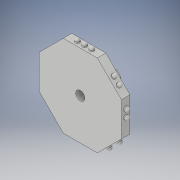
# Autodesk Inventor part: Right Braille Wheel
Saved by Autodesk Inventor 2017 (Build 210142000, 142)
## iProperties
Created: 2018-02-03
Part Number: Right Braille Wheel
Material: Generic
Document SubType Name: Modeling
Designer: Russ
Density: 1 g/cm^3
Appearance: Default
Author: Russ
Autodesk Inventor part; units mm, degrees
ref_plane "YZ Plane" through (0, 0, 0) normal (1, 0, 0) x (0, 1, 0)
ref_plane "XZ Plane" through (0, 0, 0) normal (0, 1, 0) x (-1, 0, 0)
ref_plane "XY Plane" through (0, 0, 0) normal (0, 0, 1) x (1, 0, 0)
sketch "Sketch1" plane through (0, 0, 0) normal (0, 0, 1) x (1, 0, 0)
  line L0 (6, 14.4853) -> (14.4853, 6)
  line L1 (14.4853, 6) -> (14.4853, -6)
  line L2 (14.4853, -6) -> (6, -14.4853)
  line L3 (6, -14.4853) -> (-6, -14.4853)
  line L4 (-6, -14.4853) -> (-14.4853, -6)
  line L5 (-14.4853, -6) -> (-14.4853, 6)
  line L6 (-14.4853, 6) -> (-6, 14.4853)
  line L7 (-6, 14.4853) -> (6, 14.4853)
  point P0 (0, 0)
  point P1 (0, 0)
  dimension "d2" = 12
  constraints: 16 end point, 1 coincident, 17 other
  measures "d2" distance of L4.end L5.end
extrude "Extrusion1" add sketch "Sketch1" along normal blind 3
sketch "Sketch2" plane through (-6, 14.4853, 0) normal (0, 1, 0) x (1, 0, 0)
  circle A0 centre (3.4656, -1.4986) radius 0.8
  circle A1 centre (6.0056, -1.4986) radius 0.8
  circle A2 centre (8.5456, -1.5014) radius 0.8
  line L0 (0, 0) -> (12, 0) projected
  line L1 (0, 0) -> (0, -3) projected
  line L2 (0, -3) -> (12, -3) projected
  line L3 (12, 0) -> (12, -3) projected
  point P0 (6, 0)
  dimension "d5" = 1.6
  dimension "d6" = 2.54
  dimension "d7" = 2.54
  dimension "d8" = 1.6
  dimension "d9" = 1.6
  dimension "d10" = 1.4986
  dimension "d24" = 1.4986
  dimension "d170" = 5.9944
  constraints: 3 centre point
  measures "d5" diameter of A0
  measures "d6" distance of A1.centre A0.centre
  measures "d7" distance of A2.centre A1.centre
  measures "d8" diameter of A1
  measures "d9" diameter of A2
  measures "d10" distance from line of L0 A1.centre
  measures "d24" distance from line of L2 A2.centre
  measures "d170" distance from line of L3 A1.centre
extrude "Extrusion2" add sketch "Sketch2" along normal blind 1.2 contours A0 | A1 | A2
fillet "Fillet1" radius 0.8 3 edges at (1.7456, 15.6853, 1.5014) (-0.7944, 15.6853, 1.4986) (-3.3344, 15.6853, 1.4986)
sketch "Sketch3" plane through (6, 14.4853, 0) normal (0.7071, 0.7071, 0) x (-0.7071, 0.7071, 0)
  circle A0 centre (-8.5456, 1.4986) radius 0.8
  circle A1 centre (-6.0056, 1.4986) radius 0.8
  circle A2 centre (-3.4656, 1.4986) radius 0.8
  line L0 (-10.0061, 2.6736) -> (-10.0061, 0)
  line L1 (-10.0061, 0) -> (0.0295, 0)
  line L2 (0, 3) -> (-12, 3) projected
  line L3 (-12, 0) -> (0, 0) projected
  line L4 (-12, 0) -> (-12, 3) projected
  point P0 (-3.9705, 2.6736)
  dimension "d25" = 1.6
  dimension "d26" = 2.54
  dimension "d27" = 2.54
  dimension "d28" = 1.6
  dimension "d29" = 1.6
  dimension "d31" = 1.4605
  dimension "d32" = 1.4986
  dimension "d34" = 0
  dimension "d35" = 1.4986
  dimension "d36" = 1.4986
  dimension "d169" = 5.9944
  constraints: 4 end point, 3 centre point
  measures "d25" diameter of A0
  measures "d26" distance of A1.centre A0.centre
  measures "d27" distance of A2.centre A1.centre
  measures "d28" diameter of A1
  measures "d29" diameter of A2
  measures "d31" distance from line of L0 A0.centre
  measures "d32" distance from line of L1 A2.centre
  measures "d34" distance between parallel lines of L3 L1
  measures "d35" distance from line of L1 A1.centre
  measures "d36" distance from line of L1 A0.centre
  measures "d169" distance from line of L4 A1.centre
sketch "Sketch4" plane through (14.4853, -6, 0) normal (1, 0, 0) x (0, 0, -1)
  circle A0 centre (-1.4986, 3.4544) radius 0.8
  circle A1 centre (-1.4986, 5.9944) radius 0.8
  circle A2 centre (-1.4986, 8.5344) radius 0.8
  line L0 (0.3264, 0) -> (0, 0)
  line L1 (0, 0) -> (0, 3.0295)
  line L2 (0, 3) -> (0, -5)
  line L3 (0, -5) -> (0, 3)
  line L4 (0, 12) -> (0, 0) projected
  line L5 (0, 0) -> (-3, 0) projected
  point P0 (0, 6)
  point P1 (0.3264, -0.9705)
  dimension "d40" = 1.6
  dimension "d41" = 2.54
  dimension "d42" = 2.54
  dimension "d43" = 1.6
  dimension "d44" = 1.6
  dimension "d46" = 1.4986
  dimension "d47" = 0
  dimension "d48" = 1.4986
  dimension "d49" = 1.4986
  dimension "d50" = 0
  dimension "d51" = 0
  dimension "d171" = 5.9944
  constraints: 8 end point, 3 centre point
  measures "d40" diameter of A0
  measures "d41" distance of A1.centre A0.centre
  measures "d42" distance of A2.centre A1.centre
  measures "d43" diameter of A1
  measures "d44" diameter of A2
  measures "d46" distance from line of L1 A2.centre
  measures "d47" distance between parallel lines of L3 L1
  measures "d48" distance from line of L1 A1.centre
  measures "d49" distance from line of L1 A0.centre
  measures "d50" distance between parallel lines of L4 L1
  measures "d51" distance between parallel lines of L5 L0
  measures "d171" distance from line of L5 A1.centre
sketch "Sketch6" plane through (-14.4853, -6, 0) normal (-1, 0, 0) x (0, 0, 1)
  circle A0 centre (1.5014, 3.4544) radius 0.8
  circle A1 centre (1.5014, 5.9944) radius 0.8
  circle A2 centre (1.5014, 8.5344) radius 0.8
  line L0 (1.3264, 0) -> (3, 0)
  line L1 (3, 0) -> (3, 4.0295)
  line L2 (3, -4) -> (3, 4)
  line L3 (0, 0) -> (0, 12) projected
  line L4 (3, 12) -> (3, 0) projected
  line L5 (0, 0) -> (3, 0) projected
  point P0 (0, 6)
  point P1 (1.3264, 0.0295)
  dimension "d70" = 1.6
  dimension "d71" = 2.54
  dimension "d72" = 2.54
  dimension "d73" = 1.6
  dimension "d74" = 1.6
  dimension "d76" = 1.4986
  dimension "d77" = 0
  dimension "d78" = 1.4986
  dimension "d79" = 1.4986
  dimension "d81" = 0
  dimension "d82" = 0
  dimension "d176" = 5.9944
  constraints: 6 end point, 3 centre point
  measures "d70" diameter of A0
  measures "d71" distance of A1.centre A0.centre
  measures "d72" distance of A2.centre A1.centre
  measures "d73" diameter of A1
  measures "d74" diameter of A2
  measures "d76" distance from line of L1 A2.centre
  measures "d77" distance between parallel lines of L2 L1
  measures "d78" distance from line of L1 A1.centre
  measures "d79" distance from line of L1 A0.centre
  measures "d81" distance between parallel lines of L1 L4
  measures "d82" distance between parallel lines of L5 L0
  measures "d176" distance from line of L0 A1.centre
sketch "Sketch7" plane through (-6, -14.4853, 3) normal (-0.7071, -0.7071, 0) x (-0.7071, 0.7071, 0)
  circle A0 centre (3.4544, 1.4986) radius 0.8
  circle A1 centre (5.9944, 1.4986) radius 0.8
  circle A2 centre (8.5344, 1.4986) radius 0.8
  line L0 (0, 1.115) -> (0, 0)
  line L1 (0, 0) -> (3.9792, 0)
  line L2 (7.9497, 0) -> (0, 0)
  line L3 (0, 2.4413) -> (0, 0)
  line L4 (0, 0) -> (12, 0) projected
  line L5 (0, 3) -> (0, 0) projected
  point P0 (6, 3)
  point P1 (3.9497, 2.4413)
  point P2 (-0.0208, 1.115)
  point P3 (3.9497, -0.5587)
  dimension "d83" = 1.6
  dimension "d84" = 2.54
  dimension "d85" = 2.54
  dimension "d86" = 1.6
  dimension "d87" = 1.6
  dimension "d89" = 1.4986
  dimension "d90" = 1.4986
  dimension "d91" = 1.4986
  dimension "d92" = 0
  dimension "d93" = 0
  dimension "d94" = 0
  dimension "d95" = 0
  dimension "d175" = 5.9944
  constraints: 8 end point, 3 centre point
  measures "d83" diameter of A0
  measures "d84" distance of A1.centre A0.centre
  measures "d85" distance of A2.centre A1.centre
  measures "d86" diameter of A1
  measures "d87" diameter of A2
  measures "d89" distance from line of L1 A2.centre
  measures "d90" distance from line of L1 A1.centre
  measures "d91" distance from line of L1 A0.centre
  measures "d92" distance between parallel lines of L1 L2
  measures "d93" distance between parallel lines of L3 L0
  measures "d94" distance between parallel lines of L4 L2
  measures "d95" distance between parallel lines of L5 L0
  measures "d175" distance from line of L3 A1.centre
sketch "Sketch8" plane through (-6, -14.4853, 0) normal (0, -1, 0) x (1, 0, 0)
  line L0 (7.9497, 0) -> (0, 0)
  line L1 (0, 0) -> (3.9792, 0)
  line L2 (0, 1.115) -> (0, 0)
  circle A0 centre (3.4544, 1.4986) radius 0.8
  circle A1 centre (8.5344, 1.4986) radius 0.8
  line L3 (0, 2.4413) -> (0, 0)
  circle A2 centre (5.9944, 1.4986) radius 0.8
  line L4 (0, 0) -> (8, 0)
  line L5 (0, 3) -> (0, 0)
  point P0 (6, 0)
  point P1 (4, 3)
  point P2 (3.9497, -0.5587)
  point P3 (-0.0208, 1.115)
  point P4 (3.9497, 2.4413)
  dimension "d96" = 1.6
  dimension "d97" = 2.54
  dimension "d98" = 2.54
  dimension "d99" = 1.6
  dimension "d100" = 1.6
  dimension "d102" = 1.4986
  dimension "d103" = 1.4986
  dimension "d104" = 1.4986
  dimension "d105" = 0
  dimension "d106" = 0
  dimension "d107" = 0
  dimension "d108" = 0
  dimension "d173" = 5.9944
  constraints: 12 end point, 3 centre point
  measures "d96" diameter of A0
  measures "d97" distance of A2.centre A0.centre
  measures "d98" distance of A1.centre A2.centre
  measures "d99" diameter of A2
  measures "d100" diameter of A1
  measures "d102" distance from line of L1 A1.centre
  measures "d103" distance from line of L1 A2.centre
  measures "d104" distance from line of L1 A0.centre
  measures "d105" distance between parallel lines of L1 L0
  measures "d106" distance between parallel lines of L3 L2
  measures "d107" distance between parallel lines of L4 L0
  measures "d108" distance between parallel lines of L5 L2
  measures "d173" distance from line of L3 A2.centre
sketch "Sketch9" plane through (14.4853, -6, 3) normal (0.7071, -0.7071, 0) x (-0.7071, -0.7071, 0)
  line L0 (7.9497, 0) -> (0, 0)
  line L1 (0, 0) -> (3.9792, 0)
  line L2 (0, 1.115) -> (0, 0)
  circle A0 centre (3.4544, 1.4986) radius 0.8
  circle A1 centre (8.5344, 1.4986) radius 0.8
  line L3 (0, 2.4413) -> (0, 0)
  circle A2 centre (5.9944, 1.4986) radius 0.8
  line L4 (0, 0) -> (8, 0)
  line L5 (0, 3) -> (0, 0)
  point P0 (6, 3)
  point P1 (4, 3)
  point P2 (3.9497, -0.5587)
  point P3 (-0.0208, 1.115)
  point P4 (3.9497, 2.4413)
  dimension "d109" = 1.6
  dimension "d110" = 2.54
  dimension "d111" = 2.54
  dimension "d112" = 1.6
  dimension "d113" = 1.6
  dimension "d115" = 1.4986
  dimension "d116" = 1.4986
  dimension "d117" = 1.4986
  dimension "d118" = 0
  dimension "d119" = 0
  dimension "d120" = 0
  dimension "d121" = 0
  dimension "d172" = 5.9944
  constraints: 12 end point, 3 centre point
  measures "d109" diameter of A0
  measures "d110" distance of A2.centre A0.centre
  measures "d111" distance of A1.centre A2.centre
  measures "d112" diameter of A2
  measures "d113" diameter of A1
  measures "d115" distance from line of L1 A1.centre
  measures "d116" distance from line of L1 A2.centre
  measures "d117" distance from line of L1 A0.centre
  measures "d118" distance between parallel lines of L1 L0
  measures "d119" distance between parallel lines of L3 L2
  measures "d120" distance between parallel lines of L4 L0
  measures "d121" distance between parallel lines of L5 L2
  measures "d172" distance from line of L3 A2.centre
extrude "Extrusion6" add sketch "Sketch3" along normal blind 1.2 contours A0 | A1
fillet "Fillet5" radius 0.8 2 edges at (11.6608, 10.5215, 1.4986) (13.4569, 8.7255, 1.4986)
extrude "Extrusion7" add sketch "Sketch4" along normal blind 1.2 contours A1 | A2
fillet "Fillet6" radius 0.8 2 edges at (15.6853, 2.5344, 2.2986) (15.6853, -0.0056, 2.2986)
extrude "Extrusion8" add sketch "Sketch9" along normal blind 1.2 contours A0 | A1
fillet "Fillet7" radius 0.8 2 edges at (13.4569, -8.7255, 1.5014) (9.8648, -12.3176, 1.5014)
extrude "Extrusion9" add sketch "Sketch8" along normal blind 1.2 contours A1
fillet "Fillet8" radius 0.8 1 edges at (1.7344, -15.6853, 1.4986)
extrude "Extrusion10" add sketch "Sketch7" along normal blind 1.2 contours A1
fillet "Fillet9" radius 0.8 1 edges at (-10.5215, -11.6608, 1.5014)
extrude "Extrusion11" add sketch "Sketch6" along normal blind 1.2 contours A2
fillet "Fillet10" radius 0.8 1 edges at (-15.6853, 2.5344, 0.7014)
sketch "Sketch11" plane through (0, 0, 3) normal (0, 0, 1) x (1, 0, 0)
  arc A0 (-2.0086, 7.3505) -> (2.0086, 7.3505) centre (0, 0) ccw
  line L0 (0, 7.62) -> (0, 9.525)
  line L1 (0, 9.525) -> (1.016, 9.525)
  line L2 (0, 9.525) -> (-1.016, 9.525)
  arc A1 (-1.4866, 7.4736) -> (1.4866, 7.4736) centre (0, 0) ccw
  line L3 (-1.4866, 7.4736) -> (-1.8582, 9.342)
  line L4 (-2.916, 7.04) -> (-3.6451, 8.8)
  line L5 (-4.2334, 6.3358) -> (-5.2918, 7.9197)
  line L6 (-5.3882, 5.3882) -> (-6.7352, 6.7352)
  line L7 (-6.3358, 4.2334) -> (-7.9197, 5.2918)
  line L8 (-7.04, 2.916) -> (-8.8, 3.6451)
  line L9 (-7.4736, 1.4866) -> (-9.342, 1.8582)
  line L10 (-7.62, 0) -> (-9.525, 0)
  line L11 (-7.4736, -1.4866) -> (-9.342, -1.8582)
  line L12 (-7.04, -2.916) -> (-8.8, -3.6451)
  line L13 (-6.3358, -4.2334) -> (-7.9197, -5.2918)
  line L14 (-5.3882, -5.3882) -> (-6.7352, -6.7352)
  line L15 (-4.2334, -6.3358) -> (-5.2918, -7.9197)
  line L16 (-2.916, -7.04) -> (-3.6451, -8.8)
  line L17 (-1.4866, -7.4736) -> (-1.8582, -9.342)
  line L18 (0, -7.62) -> (0, -9.525)
  line L19 (1.4866, -7.4736) -> (1.8582, -9.342)
  line L20 (2.916, -7.04) -> (3.6451, -8.8)
  line L21 (4.2334, -6.3358) -> (5.2918, -7.9197)
  line L22 (5.3882, -5.3882) -> (6.7352, -6.7352)
  line L23 (6.3358, -4.2334) -> (7.9197, -5.2918)
  line L24 (7.04, -2.916) -> (8.8, -3.6451)
  line L25 (7.4736, -1.4866) -> (9.342, -1.8582)
  line L26 (7.62, 0) -> (9.525, 0)
  line L27 (7.4736, 1.4866) -> (9.342, 1.8582)
  line L28 (7.04, 2.916) -> (8.8, 3.6451)
  line L29 (6.3358, 4.2334) -> (7.9197, 5.2918)
  line L30 (5.3882, 5.3882) -> (6.7352, 6.7352)
  line L31 (4.2334, 6.3358) -> (5.2918, 7.9197)
  line L32 (2.916, 7.04) -> (3.6451, 8.8)
  line L33 (1.4866, 7.4736) -> (1.8582, 9.342)
  arc A2 (-1.4866, 7.4736) -> (1.4866, 7.4736) centre (0, 0) ccw
  arc A3 (-1.016, 9.525) -> (-1.6724, 8.4079) centre (-0.1056, 8.2386) ccw
  arc A4 (1.6724, 8.4079) -> (1.016, 9.525) centre (0.1056, 8.2386) ccw
  circle A5 centre (0, 0) radius 7.62
  line L34 (-1.4866, 7.4736) -> (-1.6724, 8.4079)
  line L35 (-1.016, 9.525) -> (1.016, 9.525)
  line L36 (1.6724, 8.4079) -> (1.4866, 7.4736)
  arc A6 (-1.016, 9.525) -> (-1.6724, 8.4079) centre (-0.1056, 8.2386) ccw
  arc A7 (1.6724, 8.4079) -> (1.016, 9.525) centre (0.1056, 8.2386) ccw
  dimension "d148" = 15.24
  dimension "d156" = 360
  dimension "d161" = 1.016
  dimension "d162" = 1.016
  dimension "d168" = 1.905
  constraints: 74 end point, 14 point on circle, 7 centre point, 5 symmetric about line, 4 coincident, 3 concentric, 2 collinear, 1 perpendicular, 1 point on line, 1 vertical, 101 other
  measures "d148" diameter of A0
  measures "d161" distance of L0.end L1.end
  measures "d162" distance of L0.end L2.end
  measures "d168" distance of L0.start L0.end
extrude "Extrusion14" add sketch "Sketch11" against normal blind 6.81
pattern_circular "Circular Pattern4" count 8 over 360 about axis through (0, 0, 3) along (0, 0, -1) of "Extrusion14"
sketch "Sketch12" plane through (0, 0, -3.81) normal (0, 0, -1) x (1, 0, 0)
  circle A0 centre (0, 0) radius 1.6
  dimension "d177" = 3.2
  constraints: 1 centre point, 1 coincident
  measures "d177" diameter of A0
extrude "Extrusion15" cut sketch "Sketch12" against normal up to next
body "Solid1"
